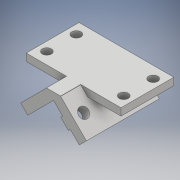
# Autodesk Inventor part: Estrutura - suporteCam
Saved by Autodesk Inventor 2017 (Build 210142000, 142)
## iProperties
Created: 2020-10-25
Part Number: Estrutura - suporteCam
Material: Generic
Document SubType Name: Modeling
Designer: ale
Density: 1 g/cm^3
Appearance: Default
Author: ale
Autodesk Inventor part; units mm, degrees
ref_plane "YZ Plane" through (0, 0, 0) normal (1, 0, 0) x (0, 1, 0)
sketch "Sketch1" plane through (0, 0, 0) normal (0, 0, 1) x (1, 0, 0)
  line L0 (-26, 14.5) -> (26, 14.5)
  line L1 (26, 14.5) -> (26, -14.5)
  line L2 (26, -14.5) -> (-26, -14.5)
  line L3 (-26, -14.5) -> (-26, 14.5)
  line L4 (-26, 14.5) -> (26, -14.5) construction
  line L5 (26, 14.5) -> (-26, -14.5) construction
  point P0 (0, 0)
  dimension "d0" = 52
  dimension "d1" = 29
  constraints: 12 end point, 2 midpoint, 2 parallel, 1 horizontal, 1 perpendicular
  measures "d0" distance of L1.end L2.end
  measures "d1" distance of L0.end L1.end
extrude "Extrusion1" add sketch "Sketch1" along normal blind 4
sketch "Sketch2" plane through (0, 0, 4) normal (0, 0, 1) x (1, 0, 0)
  line L0 (-21.1, 8.1) -> (21.1, 8.1)
  line L1 (21.1, 8.1) -> (21.1, -8.1)
  line L2 (21.1, -8.1) -> (-21.1, -8.1)
  line L3 (-21.1, -8.1) -> (-21.1, 8.1)
  line L4 (-21.1, 8.1) -> (21.1, -8.1) construction
  line L5 (21.1, 8.1) -> (-21.1, -8.1) construction
  point P0 (0, 0)
  dimension "d4" = 42.2
  dimension "d5" = 16.2
  constraints: 12 end point, 4 coincident, 2 midpoint, 2 parallel, 1 horizontal, 1 perpendicular
  measures "d4" distance of L1.end L2.end
  measures "d5" distance of L0.end L1.end
hole "Hole1" at (-21.1, 8.1, 4) at (21.1, 8.1, 4) at (21.1, -8.1, 4) at (-21.1, -8.1, 4) direction (0, 0, -1) diameter 5 end through all
ref_plane "Work Plane1" through (0, -14.5, 0) normal (1, 0, 0) x (0, 0, -1)
ref_plane "Work Plane2" through (0, 0, 0) normal (0.7071068, 0, -0.7071068) x (0, -1, 0)
ref_plane "Work Plane3" through (0, 0, 0) normal (-0.7071068, 0, -0.7071068) x (0, 1, 0)
sketch "Sketch4" plane through (0, 0, 0) normal (-0.7071068, 0, -0.7071068) x (0, 1, 0)
  line L0 (14.5, 15.5563) -> (14.5, -21.2132) projected
  line L1 (14.5, 0) -> (-25.5, 0)
  line L2 (-25.5, 0) -> (-25.5, 20)
  line L3 (-25.5, 20) -> (14.5, 20)
  line L4 (14.5, 20) -> (14.5, 0)
  point P0 (0, 0)
  dimension "d14" = 40
  dimension "d15" = 20
  constraints: 8 end point, 2 parallel, 1 horizontal, 1 perpendicular, 1 point on line
  measures "d14" distance of L2.end L3.end
  measures "d15" distance of L1.end L2.end
extrude "Extrusion2" add sketch "Sketch4" against normal blind 5.5
sketch "Sketch5" plane through (0, 0, 0) normal (0.7071068, 0, -0.7071068) x (0, -1, 0)
  line L0 (-14.5, -21.2132) -> (-14.5, 15.5563) projected
  line L1 (-14.5, 0) -> (25.5, 0)
  line L2 (25.5, 0) -> (25.5, 20)
  line L3 (25.5, 20) -> (-14.5, 20)
  line L4 (-14.5, 20) -> (-14.5, 0)
  point P0 (0, 0)
  dimension "d18" = 40
  dimension "d19" = 20
  constraints: 8 end point, 2 parallel, 1 horizontal, 1 perpendicular, 1 point on line
  measures "d18" distance of L3.end L2.end
  measures "d19" distance of L2.end L1.end
extrude "Extrusion3" add sketch "Sketch5" against normal blind 5.5
sketch "Sketch7" plane through (0, 0, 0) normal (-0.7071068, 0, -0.7071068) x (-0.7071068, 0, 0.7071068)
  line L0 (-20, 14.5) -> (0, 14.5) projected
  line L1 (-13, 14.5) -> (-13, -25.5)
  line L2 (0, -25.5) -> (-20, -25.5) projected
  line L3 (-7, 14.5) -> (-7, -25.5)
  line L4 (-20, -25.5) -> (-20, 14.5) projected
  line L5 (-13, 14.5) -> (-7, 14.5)
  line L6 (-13, -25.5) -> (-7, -25.5)
  point P0 (0, 0)
  dimension "d22" = 7
  dimension "d23" = 13
  constraints: 8 end point, 2 point on line, 2 vertical, 1 parallel, 1 perpendicular
  measures "d22" distance between parallel lines of L4 L1
  measures "d23" distance between parallel lines of L4 L3
extrude "Extrusion4" add sketch "Sketch7" along normal blind 1.5 contours L0 L3 L2 L1
sketch "Sketch8" plane through (-26, -14.5, 4) normal (0, -1, 0) x (1, 0, 0)
  line L0 (22.1109, -0.1109) -> (26, -4)
  line L1 (26, -4) -> (29.8891, -0.1109)
  line L2 (29.8891, -0.1109) -> (29.8891, 0)
  line L3 (0, 0) -> (52, 0) projected
  line L4 (22.1109, -0.1109) -> (26, -4) projected
  line L5 (22.1109, -0.1109) -> (22.1109, 0)
  line L6 (22.1109, 0) -> (29.8891, 0)
  constraints: 10 end point, 2 perpendicular, 2 vertical, 1 point on line
extrude "Extrusion5" add sketch "Sketch8" along normal blind 11
sketch "Sketch9" plane through (-1.0607, 0, -1.0607) normal (-0.7071068, 0, -0.7071068) x (-0.7071068, 0, 0.7071068)
  line L0 (-13, -25.5) -> (-7, -25.5) projected
  line L1 (-20, -25.5) -> (-20, 14.5) projected
  point P0 (0, 0)
  point P1 (-10, -20)
  dimension "d28" = 5.5
  dimension "d29" = 10
  measures "d28" distance from line of L0 point (-10, -20)
  measures "d29" distance from line of L1 point (-10, -20)
hole "Hole2" at (6.0104, -20, -8.1317) direction (0.7071068, 0, 0.7071068) diameter 5.5 end through all counterbore diameter 10 counterbore depth 1.5
sketch "Sketch10" plane through (0, 0, 0) normal (0.7071068, 0, -0.7071068) x (-0.7071068, 0, -0.7071068)
  line L0 (20, -25.5) -> (20, 14.5) projected
  line L1 (0, -25.5) -> (20, -25.5) projected
  point P0 (0, 0)
  point P1 (10, -20)
  dimension "d37" = 10
  dimension "d38" = 5.5
  measures "d37" distance from line of point (10, -20) L0
  measures "d38" distance from line of L1 point (10, -20)
hole "Hole3" at (-7.0711, -20, -7.0711) direction (-0.7071068, 0, 0.7071068) diameter 5.5 end through all
body "Solid1"
